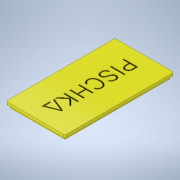
# Autodesk Inventor part: Receiver Lid
Saved by Autodesk Inventor 2020.1 (Build 241239000, 239)
## iProperties
Created: 2019-07-15
Part Number: Receiver Lid
Material: Generic
Document SubType Name: Modeling
Designer: Petar
Density: 1 g/cm^3
Appearance: Yellow
Author: Petar
Autodesk Inventor part; units mm, degrees
ref_plane "YZ Plane" through (0, 0, 0) normal (1, 0, 0) x (0, 1, 0)
ref_plane "XZ Plane" through (0, 0, 0) normal (0, 1, 0) x (-1, 0, 0)
ref_plane "XY Plane" through (0, 0, 0) normal (0, 0, 1) x (1, 0, 0)
derived "Receiver Case.ipt"
sketch "Sketch1_1" plane through (0, 0, 0) normal (0, 1, 0) x (-1, 0, 0)
  line L0 (-19.7, 38.3) -> (19.7, 38.3)
  line L1 (20.7, 37.3) -> (20.7, -37.3)
  line L2 (19.7, -38.3) -> (-19.7, -38.3)
  line L3 (-20.7, -37.3) -> (-20.7, 37.3)
  line L4 (-20.7, 38.3) -> (20.7, -38.3) construction
  line L5 (20.7, 38.3) -> (-20.7, -38.3) construction
  arc A0 (20.7, 37.3) -> (19.7, 38.3) centre (19.7, 37.3) ccw
  arc A1 (19.7, -38.3) -> (20.7, -37.3) centre (19.7, -37.3) ccw
  arc A2 (-20.7, -37.3) -> (-19.7, -38.3) centre (-19.7, -37.3) ccw
  arc A3 (-19.7, 38.3) -> (-20.7, 37.3) centre (-19.7, 37.3) ccw
  line L6 (19.5, -37.1) -> (19.5, 37.1)
  line L7 (19.5, 37.1) -> (-19.5, 37.1)
  line L8 (-19.5, 37.1) -> (-19.5, -37.1)
  line L9 (-19.5, -37.1) -> (19.5, -37.1)
  arc A4 (19.4, 36.1265) -> (18.7515, 36.775) centre (18.7515, 36.1265) ccw
  arc A5 (18.7515, -36.775) -> (19.4, -36.1265) centre (18.7515, -36.1265) ccw
  arc A6 (-19.4, -36.1265) -> (-18.7515, -36.775) centre (-18.7515, -36.1265) ccw
  arc A7 (-18.7515, 36.775) -> (-19.4, 36.1265) centre (-18.7515, 36.1265) ccw
  line L10 (0, 6.7) -> (-18.3, 6.7)
  line L11 (19.5, 35.9) -> (-9.75, 35.9)
  line L12 (-18.3, 6.7) -> (-18.3, -37.1)
  line L13 (-18.8515, -37.1) -> (0, -37.1)
  line L14 (0, -37.1) -> (0, 6.7)
  line L15 (-9.75, 35.9) -> (-9.75, 20.4)
  line L16 (-9.75, 20.4) -> (19.5, 20.4)
  line L17 (19.5, 20.4) -> (19.5, 35.9)
  circle A8 centre (-15.1037, 23.0728) radius 1.75
  line L18 (-11.8537, 34.3228) -> (-18.3537, 34.3228)
  line L19 (-18.3537, 34.3228) -> (-18.3537, 27.8228)
  line L20 (-18.3537, 27.8228) -> (-11.8537, 27.8228)
  line L21 (-11.8537, 27.8228) -> (-11.8537, 34.3228)
  line L22 (-11.8537, 34.3228) -> (-18.3537, 27.8228) construction
  line L23 (-18.3537, 34.3228) -> (-11.8537, 27.8228) construction
  circle A9 centre (-15.1037, 31.0728) radius 2
  line L24 (18.3, 18.9) -> (1.5, 18.9)
  line L25 (1.5, 18.9) -> (1.5, -37.1)
  line L26 (1.5, -37.1) -> (18.3, -37.1)
  line L27 (18.3, -37.1) -> (18.3, 18.9)
  line L28 (-15.1037, 23.0728) -> (-15.1037, 31.0728) construction
  line L29 (18.3, 1.1) -> (1.5, 1.1) construction
  line L30 (-15.1037, 34.3228) -> (-15.1037, 27.8228) construction
  line L31 (-18.3537, 34.3228) -> (-11.8537, 34.3228)
  point P0 (0, 0)
  point P1 (0, 0)
sketch "Sketch3" plane through (0, 0, 0) normal (0, 1, 0) x (-1, 0, 0)
  line L0 (20.7, 37.3) -> (20.7, -37.3) projected
  arc A0 (20.7, 37.3) -> (19.7, 38.3) centre (19.7, 37.3) ccw projected
  line L1 (-19.7, 38.3) -> (19.7, 38.3) projected
  line L2 (-20.7, -37.3) -> (-20.7, 37.3) projected
  arc A1 (-20.7, -37.3) -> (-19.7, -38.3) centre (-19.7, -37.3) ccw projected
  line L3 (19.7, -38.3) -> (-19.7, -38.3) projected
  arc A2 (19.7, -38.3) -> (20.7, -37.3) centre (19.7, -37.3) ccw projected
  line L4 (19.5, -37.1) -> (19.5, 37.1) construction
  line L5 (-19.5, -37.1) -> (19.5, -37.1) construction
  line L6 (-19.5, 37.1) -> (-19.5, -37.1) construction
  line L7 (19.5, 37.1) -> (-19.5, 37.1) construction
  line L8 (18.55, 35.75) -> (18.55, -35.75)
  line L9 (18.15, -36.15) -> (-18.15, -36.15)
  line L10 (-18.55, -35.75) -> (-18.55, 35.75)
  line L11 (-18.15, 36.15) -> (18.15, 36.15)
  arc A3 (18.55, 35.75) -> (18.15, 36.15) centre (18.15, 35.75) ccw
  arc A4 (-18.15, 36.15) -> (-18.55, 35.75) centre (-18.15, 35.75) ccw
  arc A5 (-18.55, -35.75) -> (-18.15, -36.15) centre (-18.15, -35.75) ccw
  arc A6 (18.15, -36.15) -> (18.55, -35.75) centre (18.15, -35.75) ccw
  arc A7 (-19.7, 38.3) -> (-20.7, 37.3) centre (-19.7, 37.3) ccw projected
  line L12 (-19.35, 36.95) -> (19.35, 36.95)
  line L13 (19.35, 36.95) -> (19.35, -36.95)
  line L14 (19.35, -36.95) -> (-19.35, -36.95)
  line L15 (-19.35, -36.95) -> (-19.35, 36.95)
  point P0 (0, 0)
  dimension "d8" = 0.4
  dimension "d15" = 0.15
  dimension "d16" = 0.15
  dimension "d17" = 0.15
  dimension "d18" = 0.15
  dimension "d19" = 0.8
  constraints: 16 end point, 8 point on circle, 8 tangent, 4 centre point, 3 equal radius, 2 parallel, 1 horizontal, 1 perpendicular, 3 other
  measures "d8" radius of A3
  measures "d15" distance between parallel lines of L5 L14
  measures "d16" distance between parallel lines of L4 L13
  measures "d17" distance between parallel lines of L15 L6
  measures "d18" distance between parallel lines of L12 L7
  measures "d19" distance between parallel lines of L8 L13
extrude "Extrusion3" add sketch "Sketch3" along normal blind 2 contours L0 A2 L3 A1 L2 A7 L1 A0 | L8 A6 L9 A5 L10 A4 L11 A3 | L12 L13 L14 L15
extrude "Extrusion4" add sketch "Sketch3" against normal blind 2 contours L12 L13 L14 L15
sketch "Sketch4" plane through (0, 2, 0) normal (0, 1, 0) x (1, 0, 0)
  line L0 (-0.7675, 27.9872) -> (-0.7675, 27.0699)
  spline S0 degree 3 poles (-0.7675, 27.0699) (-0.7675, 25.6449) (-0.6733, 24.8545) (-0.4231, 24.1584) knots 0 0 0 0 1 1 1 1
  line L1 (4.8598, 28.8575) -> (-5.0823, 28.8575)
  line L2 (-5.0823, 20.0829) -> (-5.0823, 19.2127)
  line L3 (-5.0823, 27.9872) -> (-0.7675, 27.9872)
  line L4 (-5.0823, 28.8575) -> (-5.0823, 27.9872)
  line L5 (0.0664, 26.8342) -> (0.0664, 27.9872)
  spline S1 degree 3 poles (0.3782, 24.336) (0.1135, 24.869) (0.0664, 25.2534) (0.0664, 26.8342) knots 0 0 0 0 1 1 1 1
  spline S2 degree 3 poles (2.2419, 23.3933) (1.35, 23.3389) (0.7046, 23.6652) (0.3782, 24.336) knots 0 0 0 0 1 1 1 1
  line L6 (0.0664, 27.9872) -> (4.0258, 27.9872)
  spline S3 degree 3 poles (4.0113, 26.4898) (3.9968, 25.0974) (3.9896, 24.9778) (3.9171, 24.7131) knots 0 0 0 0 1 1 1 1
  spline S4 degree 3 poles (1.4043, 22.4905) (1.8249, 22.4071) (2.6118, 22.4361) (3.0033, 22.5485) knots 0 0 0 0 1 1 1 1
  spline S5 degree 3 poles (3.9171, 24.7131) (3.6778, 23.8393) (3.1846, 23.4549) (2.2419, 23.3933) knots 0 0 0 0 1 1 1 1
  spline S6 degree 3 poles (3.0033, 22.5485) (3.986, 22.8313) (4.5117, 23.5021) (4.7474, 24.7711) knots 0 0 0 0 1 1 1 1
  spline S7 degree 3 poles (-0.4231, 24.1584) (-0.0968, 23.241) (0.5341, 22.6645) (1.4043, 22.4905) knots 0 0 0 0 1 1 1 1
  line L7 (-2.7908, 15.4672) -> (-2.5079, 15.5252)
  spline S8 degree 3 poles (-3.7335, 15.0357) (-3.5087, 15.217) (-3.1135, 15.3983) (-2.7908, 15.4672) knots 0 0 0 0 1 1 1 1
  spline S9 degree 3 poles (-4.4514, 13.7159) (-4.4011, 13.9826) (-4.317, 14.2453) (-4.0721, 14.6957) (-3.9221, 14.8848) (-3.7335, 15.0357) knots -1.494677 -1.494677 -1.494677 -1.494677 -0.705114 -0.705114 0 0 0 0
  line L8 (-2.5079, 16.4607) -> (-2.6784, 16.4353)
  line L9 (-2.5079, 15.5252) -> (-2.5079, 16.4607)
  spline S10 degree 3 poles (-2.6784, 16.4353) (-3.2005, 16.3591) (-3.8459, 16.0945) (-4.2048, 15.8044) knots 0 0 0 0 1 1 1 1
  spline S11 degree 3 poles (-4.2048, 15.8044) (-4.9155, 15.2315) (-5.2998, 14.2344) (-5.2998, 12.9581) knots 0 0 0 0 1 1 1 1
  line L10 (4.8525, 20.0829) -> (-5.0823, 20.0829)
  line L11 (-5.0823, 19.2127) -> (4.8525, 19.2127)
  spline S12 degree 3 poles (2.2419, 16.2286) (1.4225, 16.1815) (0.8351, 15.8334) (0.3565, 15.1046) knots 0 0 0 0 1 1 1 1
  spline S13 degree 3 poles (0.3782, 13.0125) (0.4822, 13.3043) (0.6024, 13.6153) (0.8169, 14.086) (0.9303, 14.3131) (1.049, 14.4846) knots -1.508252 -1.508252 -1.508252 -1.508252 -0.608749 -0.608749 0 0 0 0
  spline S14 degree 3 poles (3.239, 15.1481) (3.6886, 14.9813) (4.073, 14.4773) (4.2216, 13.8646) knots 0 0 0 0 1 1 1 1
  spline S15 degree 3 poles (4.9976, 13.9552) (4.7583, 15.4237) (3.685, 16.312) (2.2419, 16.2286) knots 0 0 0 0 1 1 1 1
  spline S16 degree 3 poles (5.052, 13.6289) (5.0447, 13.6579) (5.0193, 13.8065) (4.9976, 13.9552) knots 0 0 0 0 1 1 1 1
  spline S17 degree 3 poles (4.2216, 13.8646) (4.3087, 13.5201) (4.305, 12.7043) (4.2216, 12.3054) knots 0 0 0 0 1 1 1 1
  line L12 (2.9381, 10.9349) -> (2.7133, 10.8914)
  line L13 (2.7133, 10.8914) -> (2.7133, 9.9994)
  line L14 (2.7133, 9.9994) -> (2.8511, 10.0248)
  spline S18 degree 3 poles (4.2216, 12.3054) (4.0548, 11.5331) (3.6125, 11.0654) (2.9381, 10.9349) knots 0 0 0 0 1 1 1 1
  spline S19 degree 3 poles (2.8511, 10.0248) (3.5291, 10.1408) (3.8953, 10.3076) (4.2579, 10.6702) knots 0 0 0 0 1 1 1 1
  spline S20 degree 3 poles (4.2579, 10.6702) (4.6459, 11.0618) (4.8489, 11.4751) (4.9831, 12.1568) knots 0 0 0 0 1 1 1 1
  spline S21 degree 3 poles (1.049, 14.4846) (1.553, 15.2206) (2.3797, 15.4708) (3.239, 15.1481) knots 0 0 0 0 1 1 1 1
  spline S22 degree 3 poles (4.7474, 24.7711) (4.8163, 25.1373) (4.8271, 25.3513) (4.8417, 27.0155) knots 0 0 0 0 1 1 1 1
  line L15 (4.8417, 27.0155) -> (4.8598, 28.8575)
  line L16 (4.0258, 27.9872) -> (4.0113, 26.4898)
  line L17 (4.8525, 19.2127) -> (4.8525, 20.0829)
  spline S23 degree 3 poles (4.9831, 12.1568) (5.0338, 12.4215) (5.0846, 13.4947) (5.052, 13.6289) knots 0 0 0 0 1 1 1 1
  spline S24 degree 3 poles (-4.4115, 12.0553) (-4.5058, 12.3888) (-4.5275, 13.3098) (-4.4514, 13.7159) knots 0 0 0 0 1 1 1 1
  spline S25 degree 3 poles (0.3565, 15.1046) (0.1027, 14.7203) (-0.104, 14.2453) (-0.463, 13.2119) knots 0 0 0 0 1 1 1 1
  ellipse E0 centre (50.9182, 62.5644) end of major axis (-4.4555, 10.3956) minor radius 14.1553 (-5.2998, 12.9581) -> (-4.93, 11.0908) ccw
  spline S26 degree 3 poles (-4.93, 11.0908) (-4.8104, 10.8442) (-4.7233, 10.7246) (-4.4877, 10.4889) knots 0 0 0 0 1 1 1 1
  spline S27 degree 3 poles (-2.74, 10.7391) (-3.6428, 10.7971) (-4.1795, 11.2213) (-4.4115, 12.0553) knots 0 0 0 0 1 1 1 1
  spline S28 degree 3 poles (-4.4877, 10.4889) (-4.0127, 10.0139) (-3.5558, 9.8326) (-2.74, 9.7964) knots 0 0 0 0 1 1 1 1
  spline S29 degree 3 poles (-0.463, 13.2119) (-0.7929, 12.2583) (-0.9343, 11.9211) (-1.1446, 11.5839) knots 0 0 0 0 1 1 1 1
  spline S30 degree 3 poles (-0.2708, 11.3627) (-0.1113, 11.6818) (0.012, 12.0009) (0.3782, 13.0125) knots 0 0 0 0 1 1 1 1
  spline S31 degree 3 poles (-2.74, 9.7964) (-2.3665, 9.7819) (-2.207, 9.7891) (-1.9894, 9.8362) knots 0 0 0 0 1 1 1 1
  spline S32 degree 3 poles (-1.9894, 9.8362) (-1.2425, 10.003) (-0.7095, 10.478) (-0.2708, 11.3627) knots 0 0 0 0 1 1 1 1
  spline S33 degree 3 poles (-1.1446, 11.5839) (-1.5362, 10.953) (-2.033, 10.6919) (-2.74, 10.7391) knots 0 0 0 0 1 1 1 1
  spline S34 degree 3 poles (2.8656, 7.0117) (1.611, 7.6317) (-0.1258, 7.813) (-1.7139, 7.4867) knots 0 0 0 0 1 1 1 1
  spline S35 degree 3 poles (-4.3644, 4.325) (-3.9329, 5.8297) (-2.3702, 6.7035) (-0.1149, 6.7035) knots 0 0 0 0 1 1 1 1
  spline S36 degree 3 poles (-4.4478, 3.4765) (-4.4478, 3.9515) (-4.4333, 4.082) (-4.3644, 4.325) knots 0 0 0 0 1 1 1 1
  spline S37 degree 3 poles (-1.7139, 7.4867) (-4.0852, 6.9972) (-5.3977, 5.4345) (-5.2853, 3.2408) knots 0 0 0 0 1 1 1 1
  spline S38 degree 3 poles (-4.1722, 2.1639) (-4.3934, 2.6063) (-4.4478, 2.8601) (-4.4478, 3.4765) knots 0 0 0 0 1 1 1 1
  spline S39 degree 3 poles (-2.8597, 1.1777) (-3.4398, 1.3046) (-3.922, 1.6708) (-4.1722, 2.1639) knots 0 0 0 0 1 1 1 1
  spline S40 degree 3 poles (-5.2853, 3.2408) (-5.2273, 2.0733) (-4.7523, 1.1233) (-3.9728, 0.6121) knots 0 0 0 0 1 1 1 1
  line L18 (-2.7618, 1.156) -> (-2.8597, 1.1777)
  spline S41 degree 3 poles (-0.1149, 6.7035) (2.144, 6.7035) (3.7031, 5.8297) (4.1346, 4.325) knots 0 0 0 0 1 1 1 1
  spline S42 degree 3 poles (5.0157, 4.1727) (4.809, 5.449) (4.0766, 6.4134) (2.8656, 7.0117) knots 0 0 0 0 1 1 1 1
  spline S43 degree 3 poles (4.218, 3.4765) (4.218, 2.987) (4.2071, 2.8782) (4.1346, 2.6426) knots 0 0 0 0 1 1 1 1
  spline S44 degree 3 poles (4.9649, 2.512) (5.0628, 2.9072) (5.0882, 3.7412) (5.0157, 4.1727) knots 0 0 0 0 1 1 1 1
  spline S45 degree 3 poles (3.743, 0.6121) (4.3449, 1.0073) (4.751, 1.6346) (4.9649, 2.512) knots 0 0 0 0 1 1 1 1
  spline S46 degree 3 poles (4.1346, 4.325) (4.2035, 4.082) (4.218, 3.9515) (4.218, 3.4765) knots 0 0 0 0 1 1 1 1
  line L19 (2.6335, 1.1777) -> (2.532, 1.156)
  line L20 (2.532, 0.2024) -> (2.7205, 0.2277)
  line L21 (2.532, 1.156) -> (2.532, 0.2024)
  spline S47 degree 3 poles (2.7205, 0.2277) (3.036, 0.2713) (3.4711, 0.4344) (3.743, 0.6121) knots 0 0 0 0 1 1 1 1
  spline S48 degree 3 poles (4.1346, 2.6426) (3.8736, 1.8231) (3.3841, 1.3445) (2.6335, 1.1777) knots 0 0 0 0 1 1 1 1
  line L22 (4.8525, -3.2313) -> (4.8525, -2.3611)
  line L23 (4.8525, -2.3611) -> (-5.0823, -2.3611)
  line L24 (-5.0823, -3.2313) -> (-0.3324, -3.2313)
  line L25 (0.5015, -3.2313) -> (4.8525, -3.2313)
  line L26 (-0.3324, -3.2313) -> (-0.3324, -8.5613)
  line L27 (4.8525, -9.4315) -> (4.8525, -8.5613)
  line L28 (4.8525, -13.6375) -> (4.8525, -12.7673)
  line L29 (4.8525, -8.5613) -> (0.5015, -8.5613)
  line L30 (0.5015, -8.5613) -> (0.5015, -3.2313)
  spline S49 degree 3 poles (-4.9083, -19.3627) (-4.814, -19.2685) (-3.7262, -18.2605) (-2.4898, -17.1183) knots 0 0 0 0 1 1 1 1
  line L31 (-5.0823, -19.5259) -> (-4.9083, -19.3627)
  line L32 (-5.0823, -18.9131) -> (-5.0823, -19.5259)
  line L33 (-5.0787, -18.2967) -> (-5.0823, -18.9131)
  spline S50 degree 3 poles (-3.9728, 0.6121) (-3.7008, 0.4344) (-3.2694, 0.2749) (-2.9503, 0.2314) knots 0 0 0 0 1 1 1 1
  line L34 (-2.9503, 0.2314) -> (-2.7618, 0.206)
  line L35 (-5.0823, -2.3611) -> (-5.0823, -3.2313)
  line L36 (-2.7618, 0.206) -> (-2.7618, 1.156)
  spline S51 degree 3 poles (4.7728, -23.895) (4.7256, -23.8769) (2.4957, -23.0067) (-0.1874, -21.9588) knots 0 0 0 0 1 1 1 1
  spline S52 degree 3 poles (1.2231, -23.3475) (3.9968, -24.4099) (4.0258, -24.4244) (3.9062, -24.4715) knots 0 0 0 0 1 1 1 1
  spline S53 degree 3 poles (4.8525, -24.4389) (4.8525, -23.9494) (4.8489, -23.9313) (4.7728, -23.895) knots 0 0 0 0 1 1 1 1
  line L37 (4.8525, -24.9429) -> (4.8525, -24.4389)
  line L38 (4.1564, -25.2185) -> (4.8525, -24.9429)
  spline S54 degree 3 poles (3.9062, -24.4715) (3.8409, -24.5006) (2.1948, -25.1206) (0.2477, -25.8566) knots 0 0 0 0 1 1 1 1
  spline S55 degree 3 poles (-0.8038, -27.1583) (1.5385, -26.241) (3.772, -25.3708) (4.1564, -25.2185) knots 0 0 0 0 1 1 1 1
  line L39 (-0.3324, -8.5613) -> (-5.0823, -8.5613)
  line L40 (-5.0823, -8.5613) -> (-5.0823, -9.4315)
  line L41 (-5.0823, -9.4315) -> (4.8525, -9.4315)
  line L42 (-5.0823, -13.6375) -> (-2.6385, -13.6448)
  spline S56 degree 3 poles (-2.4898, -17.1183) (-1.2534, -15.9762) (-0.1656, -14.9682) (-0.075, -14.8812) knots 0 0 0 0 1 1 1 1
  line L43 (-5.0823, -12.7673) -> (-5.0823, -13.6375)
  line L44 (-0.191, -13.6556) -> (-5.0787, -18.2967)
  line L45 (-2.6385, -13.6448) -> (-0.191, -13.6556)
  line L46 (4.8525, -12.7673) -> (-5.0823, -12.7673)
  line L47 (0.0882, -14.7216) -> (2.4522, -16.9008)
  line L48 (0.2259, -13.6556) -> (2.5392, -13.6448)
  spline S57 degree 3 poles (4.8344, -19.0763) (4.8453, -19.0763) (4.8525, -18.8333) (4.8525, -18.5397) knots 0 0 0 0 1 1 1 1
  spline S58 degree 3 poles (2.4522, -16.9008) (3.7539, -18.0973) (4.8271, -19.0763) (4.8344, -19.0763) knots 0 0 0 0 1 1 1 1
  line L49 (4.8525, -18.5397) -> (4.8525, -17.9994)
  line L50 (4.8525, -17.9994) -> (0.2259, -13.6556)
  line L51 (2.5392, -13.6448) -> (4.8525, -13.6375)
  line L52 (-0.075, -14.8812) -> (0.0882, -14.7216)
  spline S59 degree 3 poles (-2.091, -22.0894) (-1.8118, -22.1873) (-0.3216, -22.7565) (1.2231, -23.3475) knots 0 0 0 0 1 1 1 1
  spline S60 degree 3 poles (0.2477, -25.8566) (-1.6958, -26.5927) (-3.4978, -27.2743) (-3.7589, -27.3722) knots 0 0 0 0 1 1 1 1
  line L53 (-4.2411, -25.4578) -> (-4.2484, -23.3657)
  line L54 (-0.1874, -21.9588) -> (-5.0642, -20.0625)
  spline S61 degree 3 poles (-5.0678, -20.9508) (-5.0424, -20.9762) (-2.6892, -21.8754) (-2.091, -22.0894) knots 0 0 0 0 1 1 1 1
  line L55 (-5.0642, -20.0625) -> (-5.075, -20.4976)
  spline S62 degree 3 poles (-5.075, -20.4976) (-5.0787, -20.7369) (-5.0787, -20.9436) (-5.0678, -20.9508) knots 0 0 0 0 1 1 1 1
  line L56 (-4.2484, -23.3657) -> (-4.6581, -23.2206)
  line L57 (-4.6581, -23.2206) -> (-5.0642, -23.0792)
  line L58 (-5.0642, -23.0792) -> (-5.075, -24.5006)
  line L59 (-3.7589, -27.3722) -> (-4.2302, -27.5535)
  line L60 (-4.2302, -27.5535) -> (-4.2411, -25.4578)
  spline S63 degree 3 poles (-5.075, -24.5006) (-5.0787, -25.2837) (-5.0787, -26.5745) (-5.075, -27.3722) knots 0 0 0 0 1 1 1 1
  line L61 (-5.0642, -28.8226) -> (-0.8038, -27.1583)
  line L62 (-5.075, -27.3722) -> (-5.0642, -28.8226)
  point P0 (0, 0)
  constraints: 126 end point, 2 vertical alignment, 194 other
emboss "Emboss1" sketch "Sketch4" operation cut depth 0.4 direction (0, -1, 0)
equation "\"d16\" = d15"
equation "\"d17\" = d15"
equation "\"d18\" = d15"
body "Solid3"
